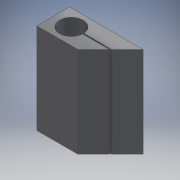
# Autodesk Inventor part: AXTSC
Saved by Autodesk Inventor 2016 (Build 200138000, 138)
## iProperties
Created: 2017-07-16
Part Number: AXTSC
Material: PC/ABS Plastic
Document SubType Name: Modeling
Designer: ludwi
Density: 0.357273 g/cm^3
Appearance: Smooth - White
Author: ludwi
Autodesk Inventor part; units mm, degrees
ref_plane "YZ Plane" through (0, 0, 0) normal (1, 0, 0) x (0, 1, 0)
ref_plane "XZ Plane" through (0, 0, 0) normal (0, 1, 0) x (-1, 0, 0)
ref_plane "XY Plane" through (0, 0, 0) normal (0, 0, 1) x (1, 0, 0)
sketch "Sketch1" plane through (0, 0, 0) normal (0, 0, 1) x (1, 0, 0)
  line L0 (66, 18) -> (-30, 18) construction
  line L1 (-30, -18) -> (30, -18) construction
  line L2 (30, -18) -> (33.623, -14.377) construction
  line L3 (47.5, -0.5) -> (33.623, -14.377) construction
  line L4 (-30, 18) -> (-30, -18)
  line L5 (-30, -18) -> (30, -18)
  line L6 (30, -18) -> (47.5, -0.5)
  line L7 (47.5, -0.5) -> (12.9904, -0.5)
  line L8 (12.9904, 0.5) -> (48.5, 0.5)
  line L9 (48.5, 0.5) -> (66, 18)
  line L10 (66, 18) -> (-30, 18)
  arc A0 (12.9904, 0.5) -> (12.9904, -0.5) centre (0, 0) ccw
  line L11 (12.9904, 0.5) -> (12.9904, -0.5) construction
  point P0 (-30, 0)
  point P1 (18, 18)
  dimension "d2" = 36
  dimension "d4" = 60
  dimension "d5" = 135
  dimension "d7" = 13
  dimension "d10" = 1
  dimension "d12" = 30
  constraints: 24 end point, 4 collinear, 4 horizontal, 2 midpoint, 2 point on circle, 1 centre point, 1 coincident, 1 horizontal alignment, 1 perpendicular, 1 point on line, 1 vertical
  measures "d2" distance of L1.start L0.end
  measures "d4" distance of L1.start L1.end
  measures "d5" angle of L1 L2
  measures "d7" radius of A0
  measures "d10" distance between parallel lines of L8 L7
  measures "d12" distance of point (-30, 0) A0.centre
extrude "Extrusion1" add sketch "Sketch1" along normal blind 100
sketch "Sketch2" plane through (-30, 18, 0) normal (0, 1, 0) x (1, 0, 0)
  line L0 (118, 0) -> (118, -100) projected
  line L1 (118, 0) -> (2, 0) projected
  line L2 (2, -100) -> (2, 0) projected
  line L3 (2, -100) -> (118, -100) projected
  line L4 (108.825, -15) -> (108.825, -6.5) projected
  arc A0 (114.925, -6.5) -> (108.825, -6.5) centre (111.875, -6.5) ccw projected
  line L5 (114.925, -6.5) -> (114.925, -15) projected
  arc A1 (108.825, -15) -> (114.925, -15) centre (111.875, -15) ccw projected
  line L6 (5.075, -15) -> (5.075, -6.5) projected
  arc A2 (11.175, -6.5) -> (5.075, -6.5) centre (8.125, -6.5) ccw projected
  line L7 (11.175, -6.5) -> (11.175, -15) projected
  arc A3 (5.075, -15) -> (11.175, -15) centre (8.125, -15) ccw projected
  circle A4 centre (49.625, -15) radius 3.05 projected
  circle A5 centre (70.375, -15) radius 3.05 projected
  circle A6 centre (70.375, -85) radius 3.05 projected
  circle A7 centre (49.625, -85) radius 3.05 projected
  line L8 (114.925, -85) -> (114.925, -93.5) projected
  arc A8 (108.825, -93.5) -> (114.925, -93.5) centre (111.875, -93.5) ccw projected
  line L9 (108.825, -93.5) -> (108.825, -85) projected
  arc A9 (114.925, -85) -> (108.825, -85) centre (111.875, -85) ccw projected
  circle A10 centre (111.875, -57.125) radius 3.05 projected
  line L10 (67.325, -42.875) -> (67.325, -34.375) projected
  arc A11 (73.425, -34.375) -> (67.325, -34.375) centre (70.375, -34.375) ccw projected
  line L11 (73.425, -34.375) -> (73.425, -42.875) projected
  arc A12 (67.325, -42.875) -> (73.425, -42.875) centre (70.375, -42.875) ccw projected
  circle A13 centre (8.125, -42.875) radius 3.05 projected
  circle A14 centre (111.875, -42.875) radius 3.05 projected
  line L12 (46.575, -42.875) -> (46.575, -34.375) projected
  arc A15 (52.675, -34.375) -> (46.575, -34.375) centre (49.625, -34.375) ccw projected
  line L13 (52.675, -34.375) -> (52.675, -42.875) projected
  arc A16 (46.575, -42.875) -> (52.675, -42.875) centre (49.625, -42.875) ccw projected
  circle A17 centre (8.125, -57.125) radius 3.05 projected
  line L14 (46.575, -65.625) -> (46.575, -57.125) projected
  arc A18 (52.675, -57.125) -> (46.575, -57.125) centre (49.625, -57.125) ccw projected
  line L15 (52.675, -57.125) -> (52.675, -65.625) projected
  arc A19 (46.575, -65.625) -> (52.675, -65.625) centre (49.625, -65.625) ccw projected
  line L16 (5.075, -93.5) -> (5.075, -85) projected
  arc A20 (11.175, -85) -> (5.075, -85) centre (8.125, -85) ccw projected
  line L17 (11.175, -85) -> (11.175, -93.5) projected
  arc A21 (5.075, -93.5) -> (11.175, -93.5) centre (8.125, -93.5) ccw projected
  line L18 (67.325, -65.625) -> (67.325, -57.125) projected
  arc A22 (73.425, -57.125) -> (67.325, -57.125) centre (70.375, -57.125) ccw projected
  line L19 (73.425, -57.125) -> (73.425, -65.625) projected
  arc A23 (67.325, -65.625) -> (73.425, -65.625) centre (70.375, -65.625) ccw projected
  point P0 (30, 0)
extrude "Extrusion2" cut sketch "Sketch2" against normal through all contours L6 A2 L7 A3 | A4 | A7 | A13 | L12 A15 L13 A16 | A17 | L14 A18 L15 A19 | L16 A20 L17 A21
chamfer "Chamfer1" distance 2 angle 45 4 edges at (-30, 18, 50) (-30, -18, 50) (66, 18, 50) (30, -18, 50)
body "Solid1"
